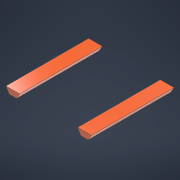
# Autodesk Inventor part: support bobine rail
Saved by Autodesk Inventor 2022 (Build 260153000, 153)
## iProperties
Created: 2022-01-17
Part Number: support bobine rail
Material: Générique
Document SubType Name: Modeling
Designer: victo
Density: 1 g/cm^3
Appearance: Par défaut
Author: victo
Autodesk Inventor part; units mm, degrees
ref_plane "YZ Plane" through (0, 0, 0) normal (1, 0, 0) x (0, 1, 0)
ref_plane "XZ Plane" through (0, 0, 0) normal (0, 1, 0) x (-1, 0, 0)
ref_plane "XY Plane" through (0, 0, 0) normal (0, 0, 1) x (1, 0, 0)
sketch "Esquisse1" plane through (0, 0, 0) normal (0, 0, 1) x (1, 0, 0)
  line L0 (-57.5, -17) -> (57.5, -17)
  line L1 (-43.0718, -17) -> (-46.5359, -11)
  line L2 (-46.5359, -11) -> (-31.5359, -11)
  line L3 (-31.5359, -11) -> (-35, -17)
  line L4 (-35, -17) -> (-43.0718, -17)
  line L5 (35, -17) -> (31.5359, -11)
  line L6 (31.5359, -11) -> (46.5359, -11)
  line L7 (46.5359, -11) -> (43.0718, -17)
  dimension "d10" = 60
  dimension "d11" = 60
  dimension "d12" = 6
  dimension "d13" = 15
  dimension "d14" = 15
  dimension "d15" = 60
  dimension "d16" = 60
  dimension "d17" = 6
  constraints: 16 end point, 3 point on line, 2 parallel, 1 horizontal
  measures "d10" angle of L1 L0
  measures "d11" angle of L0 L3
  measures "d12" distance between parallel lines of L2 L0
  measures "d13" distance of L1.end L2.end
  measures "d14" distance of L5.end L6.end
  measures "d15" angle of L0 L5
  measures "d16" angle of L0 L7
  measures "d17" distance between parallel lines of L0 L6
extrude "Extrusion1" add sketch "Esquisse1" along normal blind 90
